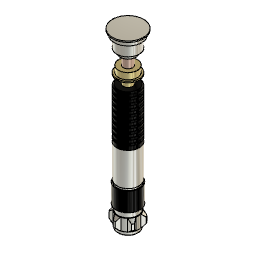
Obi Wan's Lightsaber v6 (Autodesk Fusion 360 design; units mm, degrees)
Autodesk Fusion 360 part; units mm, degrees
note: some values were not read from the file. Chosen so that the rebuilt part matches the saved one: which bodies a step acts on; which face or edge a step refers to.
sketch "Sketch1" plane through (0, 0, 0) normal (1, 0, 0) x (0, 1, 0) in component "TopCap"
ref_plane "WorkPlane1" through (0, 0, 281) normal (0, 0, 1) x (1, 0, 0) in component "TopCap"
sketch "Sketch2" plane through (0, 0, 281) normal (0, 0, 1) x (1, 0, 0) in component "TopCap"
  circle A0 centre (0, 0) radius 25
  dimension "d2" = 50
  constraint coincident A0.centre origin
  measures "d2" diameter of A0
extrude "Extrude1" add sketch "Sketch2" against normal blind 2 makes body 1 in component "TopCap"
sketch "Sketch3" plane through (0, 0, 279) normal (0, 0, -1) x (1, 0, 0) in component "TopCap"
  circle A0 centre (0, 0) radius 25
  circle A1 centre (0, 0) radius 22
  dimension "d5" = 44
  constraint coincident A0.centre A1.centre
  measures "d5" diameter of A1
extrude "Extrude2" add sketch "Sketch3" along normal blind 7 contours A1 bodies 1 in component "TopCap"
sketch "Sketch1 (2)" plane through (0, 0, 272) normal (0, 0, -1) x (1, 0, 0) in component "SecondFromTop"
  circle A0 centre (0, 0) radius 22
  circle A1 centre (0, 0) radius 18
  dimension "d8" = 36
  constraint concentric A0 A1
  measures "d8" diameter of A1
extrude "Extrude1'" add sketch "Sketch1 (2)" along normal blind 18 separate body contours A1 makes body 2 in component "SecondFromTop"
sketch "Sketch2 (2)" plane through (0, 0, 254) normal (0, 0, -1) x (1, 0, 0) in component "SecondFromTop"
  circle A0 centre (0, 0) radius 18
  circle A1 centre (0, 0) radius 12.5
  dimension "d11" = 25
  constraint coincident A0.centre A1.centre
  measures "d11" diameter of A1
extrude "Extrude2'" add sketch "Sketch2 (2)" along normal blind 7 contours A1 bodies 2 in component "SecondFromTop"
sketch "Sketch1 (3)" plane through (0, 0, 247) normal (0, 0, -1) x (1, 0, 0) in component "ThirdFromTop"
  circle A0 centre (0, 0) radius 12.5
  circle A1 centre (0, 0) radius 7.5
  dimension "d14" = 15
  constraint coincident A0.centre A1.centre
  measures "d14" diameter of A1
extrude "Extrude1''" add sketch "Sketch1 (3)" along normal blind 17 separate body contours A1 makes body 3 in component "ThirdFromTop"
sketch "Sketch2 (3)" plane through (0, 0, 230) normal (0, 0, -1) x (1, 0, 0) in component "ThirdFromTop"
  circle A0 centre (0, 0) radius 7.5
  circle A1 centre (0, 0) radius 15
  dimension "d17" = 30
  constraint coincident A0.centre A1.centre
  measures "d17" diameter of A1
extrude "Extrude2''" add sketch "Sketch2 (3)" along normal blind 10 contours A0 | A1 bodies 3 in component "ThirdFromTop"
sketch "Sketch3 (2)" plane through (0, 0, 220) normal (0, 0, -1) x (1, 0, 0) in component "ThirdFromTop"
  circle A0 centre (0, 0) radius 15
  circle A1 centre (0, 0) radius 18
  dimension "d20" = 36
  constraint concentric A0 A1
  measures "d20" diameter of A1
extrude "Extrude3" add sketch "Sketch3 (2)" along normal blind 2 contours A0 | A1 bodies 3 in component "ThirdFromTop"
sketch "Sketch4" plane through (0, 0, 218) normal (0, 0, -1) x (1, 0, 0) in component "ThirdFromTop"
  circle A0 centre (0, 0) radius 18
  circle A1 centre (0, 0) radius 12.5
  dimension "d23" = 25
  constraint coincident A0.centre A1.centre
  measures "d23" diameter of A1
extrude "Extrude4" add sketch "Sketch4" along normal blind 2 contours A1 bodies 3 in component "ThirdFromTop"
sketch "Sketch5" plane through (0, 0, 216) normal (0, 0, -1) x (1, 0, 0) in component "ThirdFromTop"
  circle A0 centre (0, 0) radius 12.5
  circle A1 centre (0, 0) radius 7.5
  dimension "d26" = 15
  constraint concentric A0 A1
  measures "d26" diameter of A1
extrude "Extrude5" add sketch "Sketch5" along normal blind 12 contours A1 bodies 3 in component "ThirdFromTop"
ref_plane "WorkPlane1" through (0, 0, 201) normal (0, 0, -1) x (1, 0, 0) in component "ThirdFromTop"
sketch "Sketch1 (4)" plane through (0, 0, 201) normal (0, 0, -1) x (1, 0, 0) in component "Grip"
cylinder "CylinderPrimitive1" add diameter 36 height 80 placed x (0, 1, 0) y (1, 0, 0) z (0, 0, -1) at (0, 0, 201) separate body makes body 4 in component "Grip"
sketch "Sketch2 (4)" plane through (0, 0, 0) normal (1, 0, 0) x (0, 1, 0) in component "Grip"
ref_plane "WorkPlane1" through (0, 0, 193) normal (0, 0, 1) x (0, -1, 0) in component "Grip"
split "Split1" by plane through (0, 0, 193) normal (0, 0, 1) bodies 4 makes body 5 at (0.6534, -10.3351, 201) in component "Grip"
chamfer "Chamfer1" distance 2 angle 45 1 edges at (6.5091, -16.7819, 201) on bodies 5 in component "Grip"
sketch "Sketch3 (3)" plane through (0, 0, 193) normal (0, 0, 1) x (1, 0, 0) in component "Grip"
chamfer "Chamfer2" distance 2 angle 45 1 edges at (6.5091, -16.7819, 193) on bodies 5 in component "Grip"
ref_plane "WorkPlane2" through (0, 0, 185) normal (0, 0, 1) x (1, 0, 0) in component "Grip"
ref_plane "WorkPlane3" through (0, 0, 177) normal (0, 0, 1) x (1, 0, 0) in component "Grip"
ref_plane "WorkPlane4" through (0, 0, 169) normal (0, 0, 1) x (1, 0, 0) in component "Grip"
ref_plane "WorkPlane5" through (0, 0, 161) normal (0, 0, 1) x (1, 0, 0) in component "Grip"
ref_plane "WorkPlane6" through (0, 0, 153) normal (0, 0, 1) x (1, 0, 0) in component "Grip"
ref_plane "WorkPlane7" through (0, 0, 145) normal (0, 0, 1) x (1, 0, 0) in component "Grip"
ref_plane "WorkPlane8" through (0, 0, 137) normal (0, 0, 1) x (1, 0, 0) in component "Grip"
ref_plane "WorkPlane9" through (0, 0, 129) normal (0, 0, 1) x (1, 0, 0) in component "Grip"
split "Split2" by plane through (0, 0, 185) normal (0, 0, 1) and through (0, 0, 177) normal (0, 0, 1) and through (0, 0, 169) normal (0, 0, 1) and through (0, 0, 161) normal (0, 0, 1) and through (0, 0, 153) normal (0, 0, 1) and through (0, 0, 145) normal (0, 0, 1) and through (0, 0, 137) normal (0, 0, 1) and through (0, 0, 129) normal (0, 0, 1) bodies 4 makes body 6 at (-1.7922, 17.9106, 166.3333) makes body 7 at (-0.8972, 17.9776, 142.3333) makes body 8 at (-0.8972, 17.9776, 131.6667) makes body 9 at (5.4781, -7.1893, 193) makes body 10 at (-0.8972, 17.9776, 182.3333) makes body 11 at (-0.8972, 17.9776, 174.3333) makes body 12 at (-0.8972, 17.9776, 158.3333) makes body 13 at (-0.8972, 17.9776, 150.3333) in component "Grip"
chamfer "Chamfer3" distance 2 angle 45 9 edges at (6.5091, -16.7819, 177) (6.5091, -16.7819, 129) (6.5091, -16.7819, 169) (6.5091, -16.7819, 161) (6.5091, -16.7819, 153) (6.5091, -16.7819, 145) (6.5091, -16.7819, 137) (6.5091, -16.7819, 193) (6.5091, -16.7819, 185) on bodies 6 7 8 9 10 12 in component "Grip"
chamfer "Chamfer4" distance 2 angle 45 6 edges at (6.5091, -16.7819, 185) (6.5091, -16.7819, 137) (6.5091, -16.7819, 161) (6.5091, -16.7819, 153) (6.5091, -16.7819, 129) (6.5091, -16.7819, 177) on bodies 4 8 10 11 12 13 in component "Grip"
chamfer "Chamfer5" distance 2 angle 45 1 edges at (6.5091, -16.7819, 169) on bodies 11 in component "Grip"
sketch "Sketch1 (5)" plane through (0, 0, 121) normal (0, 0, -1) x (1, 0, 0) in component "Handle"
  circle A0 centre (0, 0) radius 18
  circle A1 centre (0, 0) radius 19
  dimension "d46" = 38
  constraint coincident A0.centre A1.centre
  measures "d46" diameter of A1
extrude "Extrude1'''" add sketch "Sketch1 (5)" along normal blind 53 separate body contours A0 makes body 14 in component "Handle"
sketch "Sketch2 (5)" plane through (0, 0, 68) normal (0, 0, -1) x (1, 0, 0) in component "Handle"
  circle A0 centre (0, 0) radius 18
  circle A1 centre (0, 0) radius 17.5
  dimension "d49" = 35
  constraint coincident A0.centre A1.centre
  measures "d49" diameter of A1
extrude "Extrude2'''" add sketch "Sketch2 (5)" along normal blind 3 contours A1 bodies 14 in component "Handle"
sketch "Sketch3 (4)" plane through (0, 0, 65) normal (0, 0, -1) x (1, 0, 0) in component "Handle"
  circle A0 centre (0, 0) radius 17.5
  circle A1 centre (0, 0) radius 19
  dimension "d52" = 38
  constraint coincident A0.centre A1.centre
  measures "d52" diameter of A1
extrude "Extrude3'" add sketch "Sketch3 (4)" along normal blind 30 contours A0 | A1 bodies 14 in component "Handle"
sketch "Sketch1 (6)" plane through (0, 0, 35) normal (0, 0, -1) x (1, 0, 0) in component "BottomCap"
  circle A0 centre (0, 0) radius 19
  circle A1 centre (0, 0) radius 16
  dimension "d55" = 32
  constraint concentric A0 A1
  measures "d55" diameter of A1
extrude "Extrude1''''" add sketch "Sketch1 (6)" along normal blind 34 separate body contours A1 makes body 15 in component "BottomCap"
sketch "Sketch2 (6)" plane through (0, 0, 0) normal (1, 0, 0) x (0, 1, 0) in component "BottomCap"
sketch "Sketch3 (5)" plane through (0, 0, 1) normal (0, 0, -1) x (1, 0, 0) in component "BottomCap"
  circle A0 centre (0, 0) radius 16
  circle A1 centre (0, 0) radius 22 construction
  line L0 (0, -16) -> (0, -22) construction
  circle A2 centre (0, 0) radius 17
  arc A3 (0, -17) -> (4.9691, -16.2575) centre (0, 0) ccw
  line L1 (4.9691, -16.2575) -> (1.6913, -21.9349)
  line L2 (4.9691, -16.2575) -> (-1.5865, -16.2575) construction
  line L3 (-4.9691, -16.2575) -> (-1.6614, -21.9866)
  line L4 (-4.9691, -16.2575) -> (1.6463, -16.2575) construction
  arc A4 (-1.6614, -21.9866) -> (1.6913, -21.9349) centre (-0.541, 14.0544) ccw
  line L5 (16.564, -3.8254) -> (19.8418, -9.5027)
  arc A5 (18.2103, -12.4322) -> (19.8418, -9.5027) centre (-12.442, 6.5586) ccw
  line L6 (11.5949, -12.4322) -> (18.2103, -12.4322)
  circle A6 centre (0, 0) radius 17
  line L7 (11.5949, 12.4322) -> (18.1505, 12.4322)
  arc A7 (19.8717, 9.5545) -> (18.1505, 12.4322) centre (-11.9009, -7.4957) ccw
  line L8 (16.564, 3.8254) -> (19.8717, 9.5545)
  circle A8 centre (0, 0) radius 17
  line L9 (-4.9691, 16.2575) -> (-1.6913, 21.9349)
  arc A9 (1.6614, 21.9866) -> (-1.6913, 21.9349) centre (0.541, -14.0544) ccw
  line L10 (4.9691, 16.2575) -> (1.6614, 21.9866)
  circle A10 centre (0, 0) radius 17
  line L11 (-16.564, 3.8254) -> (-19.8418, 9.5027)
  arc A11 (-18.2103, 12.4322) -> (-19.8418, 9.5027) centre (12.442, -6.5586) ccw
  line L12 (-11.5949, 12.4322) -> (-18.2103, 12.4322)
  circle A12 centre (0, 0) radius 17
  line L13 (-11.5949, -12.4322) -> (-18.1505, -12.4322)
  arc A13 (-19.8717, -9.5545) -> (-18.1505, -12.4322) centre (11.9009, 7.4957) ccw
  line L14 (-16.564, -3.8254) -> (-19.8717, -9.5545)
  circle A14 centre (0, 0) radius 17
  point P0 (0, -16)
  dimension "d58" = 44
  dimension "d59" = 34
  dimension "d60" = 60
  dimension "d61" = 60
  dimension "d63" = 360
  constraint coincident A0.centre A1.centre
  constraint coincident P0 L0.start
  constraint coincident A1 L0.end
  constraint concentric A1 A2
  constraint coincident A2 A3.end
  constraint coincident A2 A3.start
  constraint coincident L0 A3.start
  constraint horizontal L2
  constraint coincident A1 L1.end
  constraint horizontal L4
  constraint coincident A2 L3.start
  constraint coincident L0.end A4
  measures "d58" diameter of A1
  measures "d59" diameter of A2
  measures "d60" angle of L1 L2
  measures "d61" angle of L3 L4
extrude "Extrude2''''" add sketch "Sketch3 (5)" along normal blind 19 separate body makes body 16 in component "BottomCap"
chamfer "Chamfer1'" distance 5 angle 45 12 edges at (-19.0601, -10.9864, -18) (-19.0601, -10.9864, 1) (-19.0446, 11.0133, 1) (-19.0446, 11.0133, -18) (0.0155, 21.9998, -18) (19.0601, 10.9864, -18) (19.0446, -11.0133, -18) (-0.0155, -21.9998, -18) (-0.0155, -21.9998, 1) (19.0446, -11.0133, 1) (19.0601, 10.9864, 1) (0.0155, 21.9998, 1) on bodies 16 in component "BottomCap"
move_body "Move1" bodies 16 to x (1, 0, 0) y (0, 1, 0) z (0, 0, 1) at (0, 0, 25) in component "BottomCap"
chamfer "Chamfer6" distance 2 angle 45 1 edges at (6.5091, -16.7819, 145) on bodies 13 in component "Grip"
fillet "Fillet1" radius 1 1 edges at (-14.9172, 5.7858, 1) on bodies 15 in component "BottomCap"
component "TopCap" placed x (1, 0, 0) y (0, 1, 0) z (0, 0, 1) at (0, 0, 0)
component "SecondFromTop" placed x (1, 0, 0) y (0, 1, 0) z (0, 0, 1) at (0, 0, 0)
component "ThirdFromTop" placed x (1, 0, 0) y (0, 1, 0) z (0, 0, 1) at (0, 0, 0)
component "Grip" placed x (1, 0, 0) y (0, 1, 0) z (0, 0, 1) at (0, 0, 3)
component "Handle" placed x (1, 0, 0) y (0, 1, 0) z (0, 0, 1) at (0, 0, 3)
component "BottomCap" placed x (1, 0, 0) y (0, 1, 0) z (0, 0, 1) at (0, 0, 3)
named bodies: "SpikyBit"
